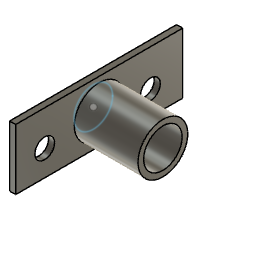
Wheel_ v2 (Autodesk Fusion 360 archive; units mm, degrees)
design "Collar"
Autodesk Fusion 360 part; units mm, degrees
sketch "Sketch1" plane through (0, 0, 0) normal (1, 0, 0) x (0, 1, 0)
  line L0 (0, 0) -> (55, 0)
  line L1 (55, 0) -> (55, 20)
  line L2 (55, 20) -> (0, 20)
  line L3 (0, 20) -> (0, 0)
  constraint horizontal L0
  constraint vertical L1
  constraint horizontal L2
  constraint vertical L3
  constraint coincident L0.start L3.end
sketch "Sketch2" plane through (0, 0, 0) normal (1, 0, 0) x (0, 1, 0)
  circle A0 centre (27.5766, 10.2067) radius 6.35
  dimension "d1" = 12.7
  measures "d1" diameter of A0
extrude "Extrude1" add sketch "Sketch1" along normal blind 2
hole "Hole1" at (2, 27.5, 10) direction (-1, 0, 0) diameter 12.7 depth 8 tip angle 118
sketch "Sketch3" plane through (2, 0, 0) normal (1, 0, 0) x (0, 1, 0)
  circle A0 centre (27.5, 10) radius 6.35
  line L0 (0, 20) -> (0, 0)
  line L1 (0, 0) -> (55, 0)
  line L2 (55, 0) -> (55, 20)
  line L3 (55, 20) -> (0, 20)
  circle A1 centre (27.5, 10) radius 8.2006
  circle A2 centre (27.5, 10) radius 6.35
  constraint concentric A0 A1
  constraint concentric A1 A2
extrude "Extrude2" add sketch "Sketch3" along normal blind 21 contours A1
hole "Hole2" at (2, 9.5562, 8.4294) direction (-1, 0, 0) diameter 6.5 depth 8 tip angle 118
hole "Hole3" at (2, 44.397, 7.8265) direction (-1, 0, 0) diameter 6.5 depth 8 tip angle 118
